Autodesk Fusion 360 part; units mm, degrees
(part 6 of 7)
sketch "Sketch2 (3)" plane through (0, 0, 43) normal (0, 0, 1) x (1, 0, 0) in component "CT idler 3"
  line L0 (67.7594, -49.5331) -> (68.0506, -49.5022)
  line L1 (68.0506, -49.5022) -> (68.1287, -49.4822)
  line L2 (68.1287, -49.4822) -> (68.2056, -49.4521)
  line L3 (68.2056, -49.4521) -> (68.2815, -49.4151)
  line L4 (68.2815, -49.4151) -> (68.3564, -49.3722)
  line L5 (68.3564, -49.3722) -> (68.4303, -49.324)
  line L6 (68.4303, -49.324) -> (68.503, -49.2708)
  line L7 (68.503, -49.2708) -> (68.5745, -49.213)
  line L8 (68.5745, -49.213) -> (68.6447, -49.1507)
  line L9 (68.6447, -49.1507) -> (68.7135, -49.0841)
  line L10 (68.7135, -49.0841) -> (68.7807, -49.0133)
  line L11 (68.7807, -49.0133) -> (68.8462, -48.9384)
  line L12 (68.8462, -48.9384) -> (68.91, -48.8596)
  line L13 (68.91, -48.8596) -> (68.8895, -48.7768)
  line L14 (68.8895, -48.7768) -> (68.8675, -48.6944)
  line L15 (68.8675, -48.6944) -> (68.8438, -48.6125)
  line L16 (68.8438, -48.6125) -> (68.7491, -48.5761)
  line L17 (68.7491, -48.5761) -> (68.6549, -48.5441)
  line L18 (68.6549, -48.5441) -> (68.5613, -48.5164)
  line L19 (68.5613, -48.5164) -> (68.4685, -48.493)
  line L20 (68.4685, -48.493) -> (68.3765, -48.4742)
  line L21 (68.3765, -48.4742) -> (68.2857, -48.4598)
  line L22 (68.2857, -48.4598) -> (68.1961, -48.4502)
  line L23 (68.1961, -48.4502) -> (68.108, -48.4454)
  line L24 (68.108, -48.4454) -> (68.0217, -48.4457)
  line L25 (68.0217, -48.4457) -> (67.9375, -48.4516)
  line L26 (67.9375, -48.4516) -> (67.8559, -48.464)
  line L27 (67.8559, -48.464) -> (67.7783, -48.4857)
  line L28 (67.7783, -48.4857) -> (67.5106, -48.6046)
  line L29 (67.5106, -48.6046) -> (67.4404, -48.4572)
  line L30 (67.4404, -48.4572) -> (67.3626, -48.3138)
  line L31 (67.3626, -48.3138) -> (67.2773, -48.1747)
  line L32 (67.2773, -48.1747) -> (67.1848, -48.0403)
  line L33 (67.1848, -48.0403) -> (67.4216, -47.868)
  line L34 (67.4216, -47.868) -> (67.4792, -47.8116)
  line L35 (67.4792, -47.8116) -> (67.5307, -47.7471)
  line L36 (67.5307, -47.7471) -> (67.578, -47.6771)
  line L37 (67.578, -47.6771) -> (67.6214, -47.6025)
  line L38 (67.6214, -47.6025) -> (67.6613, -47.5238)
  line L39 (67.6613, -47.5238) -> (67.6977, -47.4414)
  line L40 (67.6977, -47.4414) -> (67.7307, -47.3556)
  line L41 (67.7307, -47.3556) -> (67.7603, -47.2665)
  line L42 (67.7603, -47.2665) -> (67.7866, -47.1744)
  line L43 (67.7866, -47.1744) -> (67.8094, -47.0795)
  line L44 (67.8094, -47.0795) -> (67.8287, -46.9819)
  line L45 (67.8287, -46.9819) -> (67.8446, -46.8818)
  line L46 (67.8446, -46.8818) -> (67.7854, -46.8203)
  line L47 (67.7854, -46.8203) -> (67.7251, -46.76)
  line L48 (67.7251, -46.76) -> (67.6636, -46.7009)
  line L49 (67.6636, -46.7009) -> (67.5635, -46.7167)
  line L50 (67.5635, -46.7167) -> (67.4659, -46.736)
  line L51 (67.4659, -46.736) -> (67.371, -46.7588)
  line L52 (67.371, -46.7588) -> (67.2789, -46.7851)
  line L53 (67.2789, -46.7851) -> (67.1899, -46.8147)
  line L54 (67.1899, -46.8147) -> (67.104, -46.8477)
  line L55 (67.104, -46.8477) -> (67.0216, -46.8841)
  line L56 (67.0216, -46.8841) -> (66.9429, -46.924)
  line L57 (66.9429, -46.924) -> (66.8683, -46.9674)
  line L58 (66.8683, -46.9674) -> (66.7983, -47.0147)
  line L59 (66.7983, -47.0147) -> (66.7338, -47.0662)
  line L60 (66.7338, -47.0662) -> (66.6775, -47.1238)
  line L61 (66.6775, -47.1238) -> (66.5051, -47.3606)
  line L62 (66.5051, -47.3606) -> (66.3707, -47.2681)
  line L63 (66.3707, -47.2681) -> (66.2316, -47.1828)
  line L64 (66.2316, -47.1828) -> (66.0882, -47.105)
  line L65 (66.0882, -47.105) -> (65.9409, -47.0348)
  line L66 (65.9409, -47.0348) -> (66.0598, -46.7672)
  line L67 (66.0598, -46.7672) -> (66.0814, -46.6895)
  line L68 (66.0814, -46.6895) -> (66.0938, -46.6079)
  line L69 (66.0938, -46.6079) -> (66.0997, -46.5237)
  line L70 (66.0997, -46.5237) -> (66.1001, -46.4374)
  line L71 (66.1001, -46.4374) -> (66.0952, -46.3493)
  line L72 (66.0952, -46.3493) -> (66.0856, -46.2597)
  line L73 (66.0856, -46.2597) -> (66.0712, -46.1689)
  line L74 (66.0712, -46.1689) -> (66.0524, -46.0769)
  line L75 (66.0524, -46.0769) -> (66.0291, -45.9841)
  line L76 (66.0291, -45.9841) -> (66.0013, -45.8905)
  line L77 (66.0013, -45.8905) -> (65.9693, -45.7963)
  line L78 (65.9693, -45.7963) -> (65.9329, -45.7016)
  line L79 (65.9329, -45.7016) -> (65.851, -45.678)
  line L80 (65.851, -45.678) -> (65.7686, -45.6559)
  line L81 (65.7686, -45.6559) -> (65.6858, -45.6354)
  line L82 (65.6858, -45.6354) -> (65.607, -45.6992)
  line L83 (65.607, -45.6992) -> (65.5321, -45.7648)
  line L84 (65.5321, -45.7648) -> (65.4614, -45.832)
  line L85 (65.4614, -45.832) -> (65.3947, -45.9007)
  line L86 (65.3947, -45.9007) -> (65.3324, -45.9709)
  line L87 (65.3324, -45.9709) -> (65.2746, -46.0424)
  line L88 (65.2746, -46.0424) -> (65.2214, -46.1152)
  line L89 (65.2214, -46.1152) -> (65.1732, -46.189)
  line L90 (65.1732, -46.189) -> (65.1303, -46.2639)
  line L91 (65.1303, -46.2639) -> (65.0933, -46.3398)
  line L92 (65.0933, -46.3398) -> (65.0633, -46.4167)
  line L93 (65.0633, -46.4167) -> (65.0432, -46.4948)
  line L94 (65.0432, -46.4948) -> (65.0123, -46.786)
  line L95 (65.0123, -46.786) -> (64.8497, -46.7731)
  line L96 (64.8497, -46.7731) -> (64.6866, -46.7688)
  line L97 (64.6866, -46.7688) -> (64.5235, -46.7731)
  line L98 (64.5235, -46.7731) -> (64.3608, -46.786)
  line L99 (64.3608, -46.786) -> (64.33, -46.4948)
  line L100 (64.33, -46.4948) -> (64.3099, -46.4167)
  line L101 (64.3099, -46.4167) -> (64.2798, -46.3398)
  line L102 (64.2798, -46.3398) -> (64.2428, -46.2639)
  line L103 (64.2428, -46.2639) -> (64.2, -46.189)
  line L104 (64.2, -46.189) -> (64.1517, -46.1152)
  line L105 (64.1517, -46.1152) -> (64.0986, -46.0424)
  line L106 (64.0986, -46.0424) -> (64.0408, -45.9709)
  line L107 (64.0408, -45.9709) -> (63.9784, -45.9007)
  line L108 (63.9784, -45.9007) -> (63.9118, -45.832)
  line L109 (63.9118, -45.832) -> (63.841, -45.7648)
  line L110 (63.841, -45.7648) -> (63.7662, -45.6992)
  line L111 (63.7662, -45.6992) -> (63.6874, -45.6354)
  line L112 (63.6874, -45.6354) -> (63.6046, -45.6559)
  line L113 (63.6046, -45.6559) -> (63.5222, -45.678)
  line L114 (63.5222, -45.678) -> (63.4402, -45.7016)
  line L115 (63.4402, -45.7016) -> (63.4039, -45.7963)
  line L116 (63.4039, -45.7963) -> (63.3718, -45.8905)
  line L117 (63.3718, -45.8905) -> (63.3441, -45.9841)
  line L118 (63.3441, -45.9841) -> (63.3208, -46.0769)
  line L119 (63.3208, -46.0769) -> (63.3019, -46.1689)
  line L120 (63.3019, -46.1689) -> (63.2876, -46.2597)
  line L121 (63.2876, -46.2597) -> (63.2779, -46.3493)
  line L122 (63.2779, -46.3493) -> (63.2731, -46.4374)
  line L123 (63.2731, -46.4374) -> (63.2734, -46.5237)
  line L124 (63.2734, -46.5237) -> (63.2793, -46.6079)
  line L125 (63.2793, -46.6079) -> (63.2917, -46.6895)
  line L126 (63.2917, -46.6895) -> (63.3134, -46.7672)
  line L127 (63.3134, -46.7672) -> (63.4323, -47.0348)
  line L128 (63.4323, -47.0348) -> (63.285, -47.105)
  line L129 (63.285, -47.105) -> (63.1416, -47.1828)
  line L130 (63.1416, -47.1828) -> (63.0025, -47.2681)
  line L131 (63.0025, -47.2681) -> (62.8681, -47.3606)
  line L132 (62.8681, -47.3606) -> (62.6957, -47.1238)
  line L133 (62.6957, -47.1238) -> (62.6393, -47.0662)
  line L134 (62.6393, -47.0662) -> (62.5748, -47.0147)
  line L135 (62.5748, -47.0147) -> (62.5048, -46.9674)
  line L136 (62.5048, -46.9674) -> (62.4302, -46.924)
  line L137 (62.4302, -46.924) -> (62.3516, -46.8841)
  line L138 (62.3516, -46.8841) -> (62.2692, -46.8477)
  line L139 (62.2692, -46.8477) -> (62.1833, -46.8147)
  line L140 (62.1833, -46.8147) -> (62.0943, -46.7851)
  line L141 (62.0943, -46.7851) -> (62.0022, -46.7588)
  line L142 (62.0022, -46.7588) -> (61.9073, -46.736)
  line L143 (61.9073, -46.736) -> (61.8097, -46.7167)
  line L144 (61.8097, -46.7167) -> (61.7095, -46.7009)
  line L145 (61.7095, -46.7009) -> (61.648, -46.76)
  line L146 (61.648, -46.76) -> (61.5877, -46.8203)
  line L147 (61.5877, -46.8203) -> (61.5286, -46.8818)
  line L148 (61.5286, -46.8818) -> (61.5445, -46.9819)
  line L149 (61.5445, -46.9819) -> (61.5638, -47.0795)
  line L150 (61.5638, -47.0795) -> (61.5866, -47.1744)
  line L151 (61.5866, -47.1744) -> (61.6128, -47.2665)
  line L152 (61.6128, -47.2665) -> (61.6425, -47.3556)
  line L153 (61.6425, -47.3556) -> (61.6755, -47.4414)
  line L154 (61.6755, -47.4414) -> (61.7119, -47.5238)
  line L155 (61.7119, -47.5238) -> (61.7518, -47.6025)
  line L156 (61.7518, -47.6025) -> (61.7952, -47.6771)
  line L157 (61.7952, -47.6771) -> (61.8424, -47.7471)
  line L158 (61.8424, -47.7471) -> (61.894, -47.8116)
  line L159 (61.894, -47.8116) -> (61.9516, -47.868)
  line L160 (61.9516, -47.868) -> (62.1884, -48.0403)
  line L161 (62.1884, -48.0403) -> (62.0959, -48.1747)
  line L162 (62.0959, -48.1747) -> (62.0106, -48.3138)
  line L163 (62.0106, -48.3138) -> (61.9327, -48.4572)
  line L164 (61.9327, -48.4572) -> (61.8626, -48.6046)
  line L165 (61.8626, -48.6046) -> (61.5949, -48.4857)
  line L166 (61.5949, -48.4857) -> (61.5173, -48.464)
  line L167 (61.5173, -48.464) -> (61.4357, -48.4516)
  line L168 (61.4357, -48.4516) -> (61.3515, -48.4457)
  line L169 (61.3515, -48.4457) -> (61.2651, -48.4454)
  line L170 (61.2651, -48.4454) -> (61.177, -48.4502)
  line L171 (61.177, -48.4502) -> (61.0875, -48.4598)
  line L172 (61.0875, -48.4598) -> (60.9966, -48.4742)
  line L173 (60.9966, -48.4742) -> (60.9047, -48.493)
  line L174 (60.9047, -48.493) -> (60.8118, -48.5164)
  line L175 (60.8118, -48.5164) -> (60.7182, -48.5441)
  line L176 (60.7182, -48.5441) -> (60.624, -48.5761)
  line L177 (60.624, -48.5761) -> (60.5294, -48.6125)
  line L178 (60.5294, -48.6125) -> (60.5057, -48.6944)
  line L179 (60.5057, -48.6944) -> (60.4836, -48.7768)
  line L180 (60.4836, -48.7768) -> (60.4632, -48.8596)
  line L181 (60.4632, -48.8596) -> (60.527, -48.9384)
  line L182 (60.527, -48.9384) -> (60.5925, -49.0133)
  line L183 (60.5925, -49.0133) -> (60.6597, -49.0841)
  line L184 (60.6597, -49.0841) -> (60.7285, -49.1507)
  line L185 (60.7285, -49.1507) -> (60.7987, -49.213)
  line L186 (60.7987, -49.213) -> (60.8702, -49.2708)
  line L187 (60.8702, -49.2708) -> (60.9429, -49.324)
  line L188 (60.9429, -49.324) -> (61.0168, -49.3722)
  line L189 (61.0168, -49.3722) -> (61.0917, -49.4151)
  line L190 (61.0917, -49.4151) -> (61.1676, -49.4521)
  line L191 (61.1676, -49.4521) -> (61.2445, -49.4822)
  line L192 (61.2445, -49.4822) -> (61.3225, -49.5022)
  line L193 (61.3225, -49.5022) -> (61.6138, -49.5331)
  line L194 (61.6138, -49.5331) -> (61.6009, -49.6957)
  line L195 (61.6009, -49.6957) -> (61.5966, -49.8588)
  line L196 (61.5966, -49.8588) -> (61.6009, -50.0219)
  line L197 (61.6009, -50.0219) -> (61.6138, -50.1846)
  line L198 (61.6138, -50.1846) -> (61.3225, -50.2155)
  line L199 (61.3225, -50.2155) -> (61.2445, -50.2355)
  line L200 (61.2445, -50.2355) -> (61.1676, -50.2656)
  line L201 (61.1676, -50.2656) -> (61.0917, -50.3026)
  line L202 (61.0917, -50.3026) -> (61.0168, -50.3455)
  line L203 (61.0168, -50.3455) -> (60.9429, -50.3937)
  line L204 (60.9429, -50.3937) -> (60.8702, -50.4468)
  line L205 (60.8702, -50.4468) -> (60.7987, -50.5047)
  line L206 (60.7987, -50.5047) -> (60.7285, -50.567)
  line L207 (60.7285, -50.567) -> (60.6597, -50.6336)
  line L208 (60.6597, -50.6336) -> (60.5925, -50.7044)
  line L209 (60.5925, -50.7044) -> (60.527, -50.7792)
  line L210 (60.527, -50.7792) -> (60.4632, -50.858)
  line L211 (60.4632, -50.858) -> (60.4836, -50.9409)
  line L212 (60.4836, -50.9409) -> (60.5057, -51.0232)
  line L213 (60.5057, -51.0232) -> (60.5294, -51.1052)
  line L214 (60.5294, -51.1052) -> (60.624, -51.1415)
  line L215 (60.624, -51.1415) -> (60.7182, -51.1736)
  line L216 (60.7182, -51.1736) -> (60.8118, -51.2013)
  line L217 (60.8118, -51.2013) -> (60.9047, -51.2246)
  line L218 (60.9047, -51.2246) -> (60.9966, -51.2435)
  line L219 (60.9966, -51.2435) -> (61.0875, -51.2578)
  line L220 (61.0875, -51.2578) -> (61.177, -51.2675)
  line L221 (61.177, -51.2675) -> (61.2651, -51.2723)
  line L222 (61.2651, -51.2723) -> (61.3515, -51.272)
  line L223 (61.3515, -51.272) -> (61.4357, -51.2661)
  line L224 (61.4357, -51.2661) -> (61.5173, -51.2537)
  line L225 (61.5173, -51.2537) -> (61.5949, -51.232)
  line L226 (61.5949, -51.232) -> (61.8626, -51.1131)
  line L227 (61.8626, -51.1131) -> (61.9327, -51.2604)
  line L228 (61.9327, -51.2604) -> (62.0106, -51.4038)
  line L229 (62.0106, -51.4038) -> (62.0959, -51.5429)
  line L230 (62.0959, -51.5429) -> (62.1884, -51.6773)
  line L231 (62.1884, -51.6773) -> (61.9516, -51.8497)
  line L232 (61.9516, -51.8497) -> (61.894, -51.9061)
  line L233 (61.894, -51.9061) -> (61.8424, -51.9706)
  line L234 (61.8424, -51.9706) -> (61.7952, -52.0406)
  line L235 (61.7952, -52.0406) -> (61.7518, -52.1152)
  line L236 (61.7518, -52.1152) -> (61.7119, -52.1939)
  line L237 (61.7119, -52.1939) -> (61.6755, -52.2763)
  line L238 (61.6755, -52.2763) -> (61.6425, -52.3621)
  line L239 (61.6425, -52.3621) -> (61.6128, -52.4512)
  line L240 (61.6128, -52.4512) -> (61.5866, -52.5432)
  line L241 (61.5866, -52.5432) -> (61.5638, -52.6381)
  line L242 (61.5638, -52.6381) -> (61.5445, -52.7357)
  line L243 (61.5445, -52.7357) -> (61.5286, -52.8359)
  line L244 (61.5286, -52.8359) -> (61.5877, -52.8974)
  line L245 (61.5877, -52.8974) -> (61.648, -52.9577)
  line L246 (61.648, -52.9577) -> (61.7095, -53.0168)
  line L247 (61.7095, -53.0168) -> (61.8097, -53.001)
  line L248 (61.8097, -53.001) -> (61.9073, -52.9816)
  line L249 (61.9073, -52.9816) -> (62.0022, -52.9588)
  line L250 (62.0022, -52.9588) -> (62.0943, -52.9326)
  line L251 (62.0943, -52.9326) -> (62.1833, -52.903)
  line L252 (62.1833, -52.903) -> (62.2692, -52.8699)
  line L253 (62.2692, -52.8699) -> (62.3516, -52.8335)
  line L254 (62.3516, -52.8335) -> (62.4302, -52.7937)
  line L255 (62.4302, -52.7937) -> (62.5048, -52.7502)
  line L256 (62.5048, -52.7502) -> (62.5748, -52.703)
  line L257 (62.5748, -52.703) -> (62.6393, -52.6514)
  line L258 (62.6393, -52.6514) -> (62.6957, -52.5939)
  line L259 (62.6957, -52.5939) -> (62.8681, -52.3571)
  line L260 (62.8681, -52.3571) -> (63.0025, -52.4496)
  line L261 (63.0025, -52.4496) -> (63.1416, -52.5348)
  line L262 (63.1416, -52.5348) -> (63.285, -52.6127)
  line L263 (63.285, -52.6127) -> (63.4323, -52.6828)
  line L264 (63.4323, -52.6828) -> (63.3134, -52.9505)
  line L265 (63.3134, -52.9505) -> (63.2917, -53.0281)
  line L266 (63.2917, -53.0281) -> (63.2793, -53.1097)
  line L267 (63.2793, -53.1097) -> (63.2734, -53.194)
  line L268 (63.2734, -53.194) -> (63.2731, -53.2803)
  line L269 (63.2731, -53.2803) -> (63.2779, -53.3684)
  line L270 (63.2779, -53.3684) -> (63.2876, -53.4579)
  line L271 (63.2876, -53.4579) -> (63.3019, -53.5488)
  line L272 (63.3019, -53.5488) -> (63.3208, -53.6407)
  line L273 (63.3208, -53.6407) -> (63.3441, -53.7336)
  line L274 (63.3441, -53.7336) -> (63.3718, -53.8272)
  line L275 (63.3718, -53.8272) -> (63.4039, -53.9214)
  line L276 (63.4039, -53.9214) -> (63.4402, -54.016)
  line L277 (63.4402, -54.016) -> (63.5222, -54.0397)
  line L278 (63.5222, -54.0397) -> (63.6046, -54.0618)
  line L279 (63.6046, -54.0618) -> (63.6874, -54.0822)
  line L280 (63.6874, -54.0822) -> (63.7662, -54.0185)
  line L281 (63.7662, -54.0185) -> (63.841, -53.9529)
  line L282 (63.841, -53.9529) -> (63.9118, -53.8857)
  line L283 (63.9118, -53.8857) -> (63.9784, -53.8169)
  line L284 (63.9784, -53.8169) -> (64.0408, -53.7468)
  line L285 (64.0408, -53.7468) -> (64.0986, -53.6752)
  line L286 (64.0986, -53.6752) -> (64.1517, -53.6025)
  line L287 (64.1517, -53.6025) -> (64.2, -53.5286)
  line L288 (64.2, -53.5286) -> (64.2428, -53.4537)
  line L289 (64.2428, -53.4537) -> (64.2798, -53.3778)
  line L290 (64.2798, -53.3778) -> (64.3099, -53.3009)
  line L291 (64.3099, -53.3009) -> (64.33, -53.2229)
  line L292 (64.33, -53.2229) -> (64.3608, -52.9316)
  line L293 (64.3608, -52.9316) -> (64.5235, -52.9445)
  line L294 (64.5235, -52.9445) -> (64.6866, -52.9488)
  line L295 (64.6866, -52.9488) -> (64.8497, -52.9445)
  line L296 (64.8497, -52.9445) -> (65.0123, -52.9316)
  line L297 (65.0123, -52.9316) -> (65.0432, -53.2229)
  line L298 (65.0432, -53.2229) -> (65.0633, -53.3009)
  line L299 (65.0633, -53.3009) -> (65.0933, -53.3778)
  line L300 (65.0933, -53.3778) -> (65.1303, -53.4537)
  line L301 (65.1303, -53.4537) -> (65.1732, -53.5286)
  line L302 (65.1732, -53.5286) -> (65.2214, -53.6025)
  line L303 (65.2214, -53.6025) -> (65.2746, -53.6752)
  line L304 (65.2746, -53.6752) -> (65.3324, -53.7468)
  line L305 (65.3324, -53.7468) -> (65.3947, -53.8169)
  line L306 (65.3947, -53.8169) -> (65.4614, -53.8857)
  line L307 (65.4614, -53.8857) -> (65.5321, -53.9529)
  line L308 (65.5321, -53.9529) -> (65.607, -54.0185)
  line L309 (65.607, -54.0185) -> (65.6858, -54.0822)
  line L310 (65.6858, -54.0822) -> (65.7686, -54.0618)
  line L311 (65.7686, -54.0618) -> (65.851, -54.0397)
  line L312 (65.851, -54.0397) -> (65.9329, -54.016)
  line L313 (65.9329, -54.016) -> (65.9693, -53.9214)
  line L314 (65.9693, -53.9214) -> (66.0013, -53.8272)
  line L315 (66.0013, -53.8272) -> (66.0291, -53.7336)
  line L316 (66.0291, -53.7336) -> (66.0524, -53.6407)
  line L317 (66.0524, -53.6407) -> (66.0712, -53.5488)
  line L318 (66.0712, -53.5488) -> (66.0856, -53.4579)
  line L319 (66.0856, -53.4579) -> (66.0952, -53.3684)
  line L320 (66.0952, -53.3684) -> (66.1001, -53.2803)
  line L321 (66.1001, -53.2803) -> (66.0997, -53.194)
  line L322 (66.0997, -53.194) -> (66.0938, -53.1097)
  line L323 (66.0938, -53.1097) -> (66.0814, -53.0281)
  line L324 (66.0814, -53.0281) -> (66.0598, -52.9505)
  line L325 (66.0598, -52.9505) -> (65.9409, -52.6828)
  line L326 (65.9409, -52.6828) -> (66.0882, -52.6127)
  line L327 (66.0882, -52.6127) -> (66.2316, -52.5348)
  line L328 (66.2316, -52.5348) -> (66.3707, -52.4496)
  line L329 (66.3707, -52.4496) -> (66.5051, -52.3571)
  line L330 (66.5051, -52.3571) -> (66.6775, -52.5939)
  line L331 (66.6775, -52.5939) -> (66.7338, -52.6514)
  line L332 (66.7338, -52.6514) -> (66.7983, -52.703)
  line L333 (66.7983, -52.703) -> (66.8683, -52.7502)
  line L334 (66.8683, -52.7502) -> (66.9429, -52.7937)
  line L335 (66.9429, -52.7937) -> (67.0216, -52.8335)
  line L336 (67.0216, -52.8335) -> (67.104, -52.8699)
  line L337 (67.104, -52.8699) -> (67.1899, -52.903)
  line L338 (67.1899, -52.903) -> (67.2789, -52.9326)
  line L339 (67.2789, -52.9326) -> (67.371, -52.9588)
  line L340 (67.371, -52.9588) -> (67.4659, -52.9816)
  line L341 (67.4659, -52.9816) -> (67.5635, -53.001)
  line L342 (67.5635, -53.001) -> (67.6636, -53.0168)
  line L343 (67.6636, -53.0168) -> (67.7251, -52.9577)
  line L344 (67.7251, -52.9577) -> (67.7854, -52.8974)
  line L345 (67.7854, -52.8974) -> (67.8446, -52.8359)
  line L346 (67.8446, -52.8359) -> (67.8287, -52.7357)
  line L347 (67.8287, -52.7357) -> (67.8094, -52.6381)
  line L348 (67.8094, -52.6381) -> (67.7866, -52.5432)
  line L349 (67.7866, -52.5432) -> (67.7603, -52.4512)
  line L350 (67.7603, -52.4512) -> (67.7307, -52.3621)
  line L351 (67.7307, -52.3621) -> (67.6977, -52.2763)
  line L352 (67.6977, -52.2763) -> (67.6613, -52.1939)
  line L353 (67.6613, -52.1939) -> (67.6214, -52.1152)
  line L354 (67.6214, -52.1152) -> (67.578, -52.0406)
  line L355 (67.578, -52.0406) -> (67.5307, -51.9706)
  line L356 (67.5307, -51.9706) -> (67.4792, -51.9061)
  line L357 (67.4792, -51.9061) -> (67.4216, -51.8497)
  line L358 (67.4216, -51.8497) -> (67.1848, -51.6773)
  line L359 (67.1848, -51.6773) -> (67.2773, -51.5429)
  line L360 (67.2773, -51.5429) -> (67.3626, -51.4038)
  line L361 (67.3626, -51.4038) -> (67.4404, -51.2604)
  line L362 (67.4404, -51.2604) -> (67.5106, -51.1131)
  line L363 (67.5106, -51.1131) -> (67.7783, -51.232)
  line L364 (67.7783, -51.232) -> (67.8559, -51.2537)
  line L365 (67.8559, -51.2537) -> (67.9375, -51.2661)
  line L366 (67.9375, -51.2661) -> (68.0217, -51.272)
  line L367 (68.0217, -51.272) -> (68.108, -51.2723)
  line L368 (68.108, -51.2723) -> (68.1961, -51.2675)
  line L369 (68.1961, -51.2675) -> (68.2857, -51.2578)
  line L370 (68.2857, -51.2578) -> (68.3765, -51.2435)
  line L371 (68.3765, -51.2435) -> (68.4685, -51.2246)
  line L372 (68.4685, -51.2246) -> (68.5613, -51.2013)
  line L373 (68.5613, -51.2013) -> (68.6549, -51.1736)
  line L374 (68.6549, -51.1736) -> (68.7491, -51.1415)
  line L375 (68.7491, -51.1415) -> (68.8438, -51.1052)
  line L376 (68.8438, -51.1052) -> (68.8675, -51.0232)
  line L377 (68.8675, -51.0232) -> (68.8895, -50.9409)
  line L378 (68.8895, -50.9409) -> (68.91, -50.858)
  line L379 (68.91, -50.858) -> (68.8462, -50.7792)
  line L380 (68.8462, -50.7792) -> (68.7807, -50.7044)
  line L381 (68.7807, -50.7044) -> (68.7135, -50.6336)
  line L382 (68.7135, -50.6336) -> (68.6447, -50.567)
  line L383 (68.6447, -50.567) -> (68.5745, -50.5047)
  line L384 (68.5745, -50.5047) -> (68.503, -50.4468)
  line L385 (68.503, -50.4468) -> (68.4303, -50.3937)
  line L386 (68.4303, -50.3937) -> (68.3564, -50.3455)
  line L387 (68.3564, -50.3455) -> (68.2815, -50.3026)
  line L388 (68.2815, -50.3026) -> (68.2056, -50.2656)
  line L389 (68.2056, -50.2656) -> (68.1287, -50.2355)
  line L390 (68.1287, -50.2355) -> (68.0506, -50.2155)
  line L391 (68.0506, -50.2155) -> (67.7594, -50.1846)
  line L392 (67.7594, -50.1846) -> (67.7723, -50.0219)
  line L393 (67.7723, -50.0219) -> (67.7766, -49.8588)
  line L394 (67.7766, -49.8588) -> (67.7723, -49.6957)
  line L395 (67.7723, -49.6957) -> (67.7594, -49.5331)
extrude "Extrude2''" add sketch "Sketch2 (3)" along normal blind 2.4 separate body makes body 7 in component "CT idler 3"
combine "Combine1''" operation add target body 6 tool bodies 7 in component "CT idler 3"
ref_plane "WorkPlane3" through (0, 0, 41.2) normal (0, 0, 1) x (1, 0, 0) in component "CT idler 3"
sketch "Sketch3 (3)" plane through (0, 0, 41.2) normal (0, 0, 1) x (1, 0, 0) in component "CT idler 3"
  circle A0 centre (64.6866, -49.8588) radius 1.7
extrude "Extrude3''" cut sketch "Sketch3 (3)" along normal blind 4.2 bodies 6 in component "CT idler 3"
ref_plane "WorkPlane1" through (0, 0, 43.4) normal (0, 0, 1) x (1, 0, 0) in component "CT dial wheel (tool body)"
sketch "Sketch1 (5)" plane through (0, 0, 43.4) normal (0, 0, 1) x (1, 0, 0) in component "CT dial wheel (tool body)"
  line L0 (70.4894, -54.5349) -> (70.5857, -54.2102)
  line L1 (70.5857, -54.2102) -> (70.6022, -54.1307)
  line L2 (70.6022, -54.1307) -> (70.6131, -54.0495)
  line L3 (70.6131, -54.0495) -> (70.6203, -53.9673)
  line L4 (70.6203, -53.9673) -> (70.6245, -53.8842)
  line L5 (70.6245, -53.8842) -> (70.6261, -53.8004)
  line L6 (70.6261, -53.8004) -> (70.6251, -53.7159)
  line L7 (70.6251, -53.7159) -> (70.6219, -53.6308)
  line L8 (70.6219, -53.6308) -> (70.6165, -53.5452)
  line L9 (70.6165, -53.5452) -> (70.6091, -53.4591)
  line L10 (70.6091, -53.4591) -> (70.5997, -53.3725)
  line L11 (70.5997, -53.3725) -> (70.5884, -53.2855)
  line L12 (70.5884, -53.2855) -> (70.5752, -53.1981)
  line L13 (70.5752, -53.1981) -> (70.4387, -53.1625)
  line L14 (70.4387, -53.1625) -> (70.3017, -53.1286)
  line L15 (70.3017, -53.1286) -> (70.1643, -53.0965)
  line L16 (70.1643, -53.0965) -> (70.1119, -53.1677)
  line L17 (70.1119, -53.1677) -> (70.0614, -53.2393)
  line L18 (70.0614, -53.2393) -> (70.0127, -53.3115)
  line L19 (70.0127, -53.3115) -> (69.966, -53.3843)
  line L20 (69.966, -53.3843) -> (69.9213, -53.4575)
  line L21 (69.9213, -53.4575) -> (69.8788, -53.5313)
  line L22 (69.8788, -53.5313) -> (69.8386, -53.6056)
  line L23 (69.8386, -53.6056) -> (69.8009, -53.6804)
  line L24 (69.8009, -53.6804) -> (69.7658, -53.7559)
  line L25 (69.7658, -53.7559) -> (69.7339, -53.832)
  line L26 (69.7339, -53.832) -> (69.7057, -53.9089)
  line L27 (69.7057, -53.9089) -> (69.6832, -53.987)
  line L28 (69.6832, -53.987) -> (69.617, -54.3191)
  line L29 (69.617, -54.3191) -> (69.4173, -54.2815)
  line L30 (69.4173, -54.2815) -> (69.2167, -54.248)
  line L31 (69.2167, -54.248) -> (69.0156, -54.2186)
  line L32 (69.0156, -54.2186) -> (68.8139, -54.1934)
  line L33 (68.8139, -54.1934) -> (68.8523, -53.857)
  line L34 (68.8523, -53.857) -> (68.8547, -53.7758)
  line L35 (68.8547, -53.7758) -> (68.8514, -53.6939)
  line L36 (68.8514, -53.6939) -> (68.8442, -53.6117)
  line L37 (68.8442, -53.6117) -> (68.8339, -53.5291)
  line L38 (68.8339, -53.5291) -> (68.8209, -53.4463)
  line L39 (68.8209, -53.4463) -> (68.8053, -53.3633)
  line L40 (68.8053, -53.3633) -> (68.7874, -53.28)
  line L41 (68.7874, -53.28) -> (68.7672, -53.1966)
  line L42 (68.7672, -53.1966) -> (68.7449, -53.1131)
  line L43 (68.7449, -53.1131) -> (68.7206, -53.0295)
  line L44 (68.7206, -53.0295) -> (68.6944, -52.9458)
  line L45 (68.6944, -52.9458) -> (68.6662, -52.8621)
  line L46 (68.6662, -52.8621) -> (68.5256, -52.8507)
  line L47 (68.5256, -52.8507) -> (68.3848, -52.8411)
  line L48 (68.3848, -52.8411) -> (68.2439, -52.8333)
  line L49 (68.2439, -52.8333) -> (68.2047, -52.9125)
  line L50 (68.2047, -52.9125) -> (68.1674, -52.9919)
  line L51 (68.1674, -52.9919) -> (68.132, -53.0714)
  line L52 (68.132, -53.0714) -> (68.0986, -53.1511)
  line L53 (68.0986, -53.1511) -> (68.0673, -53.231)
  line L54 (68.0673, -53.231) -> (68.0382, -53.311)
  line L55 (68.0382, -53.311) -> (68.0116, -53.3912)
  line L56 (68.0116, -53.3912) -> (67.9874, -53.4715)
  line L57 (67.9874, -53.4715) -> (67.966, -53.5519)
  line L58 (67.966, -53.5519) -> (67.9478, -53.6324)
  line L59 (67.9478, -53.6324) -> (67.9334, -53.713)
  line L60 (67.9334, -53.713) -> (67.9248, -53.7938)
  line L61 (67.9248, -53.7938) -> (67.9173, -54.1324)
  line L62 (67.9173, -54.1324) -> (67.714, -54.13)
  line L63 (67.714, -54.13) -> (67.5107, -54.1318)
  line L64 (67.5107, -54.1318) -> (67.3075, -54.1379)
  line L65 (67.3075, -54.1379) -> (67.1045, -54.1481)
  line L66 (67.1045, -54.1481) -> (67.0839, -53.81)
  line L67 (67.0839, -53.81) -> (67.0722, -53.7297)
  line L68 (67.0722, -53.7297) -> (67.0547, -53.6496)
  line L69 (67.0547, -53.6496) -> (67.0334, -53.5699)
  line L70 (67.0334, -53.5699) -> (67.0089, -53.4904)
  line L71 (67.0089, -53.4904) -> (66.9816, -53.4111)
  line L72 (66.9816, -53.4111) -> (66.9519, -53.332)
  line L73 (66.9519, -53.332) -> (66.9197, -53.2532)
  line L74 (66.9197, -53.2532) -> (66.8854, -53.1745)
  line L75 (66.8854, -53.1745) -> (66.849, -53.0962)
  line L76 (66.849, -53.0962) -> (66.8105, -53.018)
  line L77 (66.8105, -53.018) -> (66.7702, -52.9402)
  line L78 (66.7702, -52.9402) -> (66.7279, -52.8626)
  line L79 (66.7279, -52.8626) -> (66.5874, -52.8758)
  line L80 (66.5874, -52.8758) -> (66.4471, -52.8908)
  line L81 (66.4471, -52.8908) -> (66.307, -52.9076)
  line L82 (66.307, -52.9076) -> (66.2821, -52.9924)
  line L83 (66.2821, -52.9924) -> (66.2591, -53.077)
  line L84 (66.2591, -53.077) -> (66.2381, -53.1615)
  line L85 (66.2381, -53.1615) -> (66.219, -53.2458)
  line L86 (66.219, -53.2458) -> (66.2021, -53.3299)
  line L87 (66.2021, -53.3299) -> (66.1874, -53.4138)
  line L88 (66.1874, -53.4138) -> (66.175, -53.4974)
  line L89 (66.175, -53.4974) -> (66.1652, -53.5806)
  line L90 (66.1652, -53.5806) -> (66.1581, -53.6635)
  line L91 (66.1581, -53.6635) -> (66.1541, -53.746)
  line L92 (66.1541, -53.746) -> (66.154, -53.8279)
  line L93 (66.154, -53.8279) -> (66.1595, -53.9089)
  line L94 (66.1595, -53.9089) -> (66.2109, -54.2437)
  line L95 (66.2109, -54.2437) -> (66.0103, -54.2766)
  line L96 (66.0103, -54.2766) -> (65.8104, -54.3137)
  line L97 (65.8104, -54.3137) -> (65.6113, -54.3549)
  line L98 (65.6113, -54.3549) -> (65.4132, -54.4003)
  line L99 (65.4132, -54.4003) -> (65.3342, -54.0709)
  line L100 (65.3342, -54.0709) -> (65.3087, -53.9938)
  line L101 (65.3087, -53.9938) -> (65.2776, -53.918)
  line L102 (65.2776, -53.918) -> (65.2427, -53.8432)
  line L103 (65.2427, -53.8432) -> (65.2048, -53.7691)
  line L104 (65.2048, -53.7691) -> (65.1642, -53.6958)
  line L105 (65.1642, -53.6958) -> (65.1212, -53.6231)
  line L106 (65.1212, -53.6231) -> (65.0759, -53.551)
  line L107 (65.0759, -53.551) -> (65.0284, -53.4795)
  line L108 (65.0284, -53.4795) -> (64.9789, -53.4087)
  line L109 (64.9789, -53.4087) -> (64.9275, -53.3384)
  line L110 (64.9275, -53.3384) -> (64.8742, -53.2688)
  line L111 (64.8742, -53.2688) -> (64.8191, -53.1997)
  line L112 (64.8191, -53.1997) -> (64.683, -53.2371)
  line L113 (64.683, -53.2371) -> (64.5475, -53.2762)
  line L114 (64.5475, -53.2762) -> (64.4124, -53.3171)
  line L115 (64.4124, -53.3171) -> (64.4026, -53.4049)
  line L116 (64.4026, -53.4049) -> (64.3947, -53.4923)
  line L117 (64.3947, -53.4923) -> (64.3886, -53.5791)
  line L118 (64.3886, -53.5791) -> (64.3845, -53.6655)
  line L119 (64.3845, -53.6655) -> (64.3825, -53.7512)
  line L120 (64.3825, -53.7512) -> (64.3825, -53.8364)
  line L121 (64.3825, -53.8364) -> (64.3849, -53.9208)
  line L122 (64.3849, -53.9208) -> (64.3896, -54.0045)
  line L123 (64.3896, -54.0045) -> (64.397, -54.0874)
  line L124 (64.397, -54.0874) -> (64.4074, -54.1693)
  line L125 (64.4074, -54.1693) -> (64.4215, -54.25)
  line L126 (64.4215, -54.25) -> (64.441, -54.3288)
  line L127 (64.441, -54.3288) -> (64.5498, -54.6496)
  line L128 (64.5498, -54.6496) -> (64.3579, -54.7168)
  line L129 (64.3579, -54.7168) -> (64.1675, -54.7881)
  line L130 (64.1675, -54.7881) -> (63.9786, -54.8632)
  line L131 (63.9786, -54.8632) -> (63.7913, -54.9423)
  line L132 (63.7913, -54.9423) -> (63.6564, -54.6317)
  line L133 (63.6564, -54.6317) -> (63.6179, -54.5602)
  line L134 (63.6179, -54.5602) -> (63.5741, -54.491)
  line L135 (63.5741, -54.491) -> (63.5268, -54.4233)
  line L136 (63.5268, -54.4233) -> (63.4766, -54.3569)
  line L137 (63.4766, -54.3569) -> (63.4239, -54.2917)
  line L138 (63.4239, -54.2917) -> (63.3688, -54.2276)
  line L139 (63.3688, -54.2276) -> (63.3117, -54.1645)
  line L140 (63.3117, -54.1645) -> (63.2525, -54.1024)
  line L141 (63.2525, -54.1024) -> (63.1915, -54.0412)
  line L142 (63.1915, -54.0412) -> (63.1287, -53.9809)
  line L143 (63.1287, -53.9809) -> (63.0641, -53.9216)
  line L144 (63.0641, -53.9216) -> (62.9978, -53.8631)
  line L145 (62.9978, -53.8631) -> (62.8703, -53.9236)
  line L146 (62.8703, -53.9236) -> (62.7436, -53.9857)
  line L147 (62.7436, -53.9857) -> (62.6177, -54.0494)
  line L148 (62.6177, -54.0494) -> (62.6233, -54.1375)
  line L149 (62.6233, -54.1375) -> (62.6307, -54.225)
  line L150 (62.6307, -54.225) -> (62.6398, -54.3115)
  line L151 (62.6398, -54.3115) -> (62.6507, -54.3973)
  line L152 (62.6507, -54.3973) -> (62.6636, -54.4821)
  line L153 (62.6636, -54.4821) -> (62.6785, -54.5659)
  line L154 (62.6785, -54.5659) -> (62.6954, -54.6487)
  line L155 (62.6954, -54.6487) -> (62.7146, -54.7303)
  line L156 (62.7146, -54.7303) -> (62.7363, -54.8106)
  line L157 (62.7363, -54.8106) -> (62.7608, -54.8895)
  line L158 (62.7608, -54.8895) -> (62.7886, -54.9665)
  line L159 (62.7886, -54.9665) -> (62.8216, -55.0408)
  line L160 (62.8216, -55.0408) -> (62.9844, -55.3377)
  line L161 (62.9844, -55.3377) -> (62.8071, -55.4373)
  line L162 (62.8071, -55.4373) -> (62.632, -55.5405)
  line L163 (62.632, -55.5405) -> (62.459, -55.6473)
  line L164 (62.459, -55.6473) -> (62.2883, -55.7577)
  line L165 (62.2883, -55.7577) -> (62.1015, -55.4752)
  line L166 (62.1015, -55.4752) -> (62.0511, -55.4115)
  line L167 (62.0511, -55.4115) -> (61.9959, -55.351)
  line L168 (61.9959, -55.351) -> (61.9376, -55.2926)
  line L169 (61.9376, -55.2926) -> (61.8767, -55.2359)
  line L170 (61.8767, -55.2359) -> (61.8134, -55.1809)
  line L171 (61.8134, -55.1809) -> (61.7481, -55.1273)
  line L172 (61.7481, -55.1273) -> (61.6809, -55.0751)
  line L173 (61.6809, -55.0751) -> (61.6118, -55.0241)
  line L174 (61.6118, -55.0241) -> (61.5411, -54.9745)
  line L175 (61.5411, -54.9745) -> (61.4687, -54.926)
  line L176 (61.4687, -54.926) -> (61.3948, -54.8788)
  line L177 (61.3948, -54.8788) -> (61.3194, -54.8327)
  line L178 (61.3194, -54.8327) -> (61.2044, -54.9144)
  line L179 (61.2044, -54.9144) -> (61.0904, -54.9976)
  line L180 (61.0904, -54.9976) -> (60.9774, -55.0821)
  line L181 (60.9774, -55.0821) -> (60.9983, -55.168)
  line L182 (60.9983, -55.168) -> (61.0207, -55.2528)
  line L183 (61.0207, -55.2528) -> (61.0447, -55.3365)
  line L184 (61.0447, -55.3365) -> (61.0704, -55.4191)
  line L185 (61.0704, -55.4191) -> (61.0978, -55.5003)
  line L186 (61.0978, -55.5003) -> (61.127, -55.5803)
  line L187 (61.127, -55.5803) -> (61.158, -55.6589)
  line L188 (61.158, -55.6589) -> (61.1911, -55.7359)
  line L189 (61.1911, -55.7359) -> (61.2264, -55.8113)
  line L190 (61.2264, -55.8113) -> (61.2642, -55.8847)
  line L191 (61.2642, -55.8847) -> (61.305, -55.9557)
  line L192 (61.305, -55.9557) -> (61.3503, -56.0231)
  line L193 (61.3503, -56.0231) -> (61.5622, -56.2873)
  line L194 (61.5622, -56.2873) -> (61.405, -56.4161)
  line L195 (61.405, -56.4161) -> (61.2504, -56.5482)
  line L196 (61.2504, -56.5482) -> (61.0986, -56.6834)
  line L197 (61.0986, -56.6834) -> (60.9497, -56.8218)
  line L198 (60.9497, -56.8218) -> (60.7166, -56.576)
  line L199 (60.7166, -56.576) -> (60.656, -56.522)
  line L200 (60.656, -56.522) -> (60.5911, -56.4719)
  line L201 (60.5911, -56.4719) -> (60.5235, -56.4246)
  line L202 (60.5235, -56.4246) -> (60.4537, -56.3794)
  line L203 (60.4537, -56.3794) -> (60.3818, -56.3361)
  line L204 (60.3818, -56.3361) -> (60.3082, -56.2947)
  line L205 (60.3082, -56.2947) -> (60.2329, -56.2549)
  line L206 (60.2329, -56.2549) -> (60.1561, -56.2168)
  line L207 (60.1561, -56.2168) -> (60.0778, -56.1802)
  line L208 (60.0778, -56.1802) -> (59.9981, -56.145)
  line L209 (59.9981, -56.145) -> (59.9171, -56.1113)
  line L210 (59.9171, -56.1113) -> (59.8349, -56.0791)
  line L211 (59.8349, -56.0791) -> (59.7358, -56.1795)
  line L212 (59.7358, -56.1795) -> (59.638, -56.2812)
  line L213 (59.638, -56.2812) -> (59.5414, -56.3841)
  line L214 (59.5414, -56.3841) -> (59.5769, -56.465)
  line L215 (59.5769, -56.465) -> (59.6136, -56.5447)
  line L216 (59.6136, -56.5447) -> (59.6518, -56.6229)
  line L217 (59.6518, -56.6229) -> (59.6914, -56.6997)
  line L218 (59.6914, -56.6997) -> (59.7325, -56.775)
  line L219 (59.7325, -56.775) -> (59.7752, -56.8487)
  line L220 (59.7752, -56.8487) -> (59.8194, -56.9207)
  line L221 (59.8194, -56.9207) -> (59.8654, -56.9908)
  line L222 (59.8654, -56.9908) -> (59.9132, -57.0589)
  line L223 (59.9132, -57.0589) -> (59.9632, -57.1246)
  line L224 (59.9632, -57.1246) -> (60.0157, -57.1874)
  line L225 (60.0157, -57.1874) -> (60.072, -57.246)
  line L226 (60.072, -57.246) -> (60.3266, -57.4694)
  line L227 (60.3266, -57.4694) -> (60.1941, -57.6235)
  line L228 (60.1941, -57.6235) -> (60.0648, -57.7804)
  line L229 (60.0648, -57.7804) -> (59.9388, -57.94)
  line L230 (59.9388, -57.94) -> (59.8162, -58.1021)
  line L231 (59.8162, -58.1021) -> (59.544, -57.9005)
  line L232 (59.544, -57.9005) -> (59.4749, -57.8579)
  line L233 (59.4749, -57.8579) -> (59.4023, -57.8198)
  line L234 (59.4023, -57.8198) -> (59.3275, -57.7849)
  line L235 (59.3275, -57.7849) -> (59.2509, -57.7525)
  line L236 (59.2509, -57.7525) -> (59.1726, -57.7224)
  line L237 (59.1726, -57.7224) -> (59.0929, -57.6944)
  line L238 (59.0929, -57.6944) -> (59.0119, -57.6683)
  line L239 (59.0119, -57.6683) -> (58.9296, -57.6441)
  line L240 (58.9296, -57.6441) -> (58.8461, -57.6216)
  line L241 (58.8461, -57.6216) -> (58.7616, -57.6009)
  line L242 (58.7616, -57.6009) -> (58.676, -57.5818)
  line L243 (58.676, -57.5818) -> (58.5893, -57.5642)
  line L244 (58.5893, -57.5642) -> (58.5092, -57.6804)
  line L245 (58.5092, -57.6804) -> (58.4305, -57.7975)
  line L246 (58.4305, -57.7975) -> (58.3533, -57.9156)
  line L247 (58.3533, -57.9156) -> (58.4022, -57.9892)
  line L248 (58.4022, -57.9892) -> (58.4523, -58.0612)
  line L249 (58.4523, -58.0612) -> (58.5035, -58.1316)
  line L250 (58.5035, -58.1316) -> (58.5559, -58.2004)
  line L251 (58.5559, -58.2004) -> (58.6094, -58.2674)
  line L252 (58.6094, -58.2674) -> (58.6642, -58.3326)
  line L253 (58.6642, -58.3326) -> (58.7202, -58.3958)
  line L254 (58.7202, -58.3958) -> (58.7777, -58.4569)
  line L255 (58.7777, -58.4569) -> (58.8366, -58.5156)
  line L256 (58.8366, -58.5156) -> (58.8973, -58.5716)
  line L257 (58.8973, -58.5716) -> (58.9599, -58.6244)
  line L258 (58.9599, -58.6244) -> (59.0255, -58.6723)
  line L259 (59.0255, -58.6723) -> (59.315, -58.848)
  line L260 (59.315, -58.848) -> (59.2113, -59.0229)
  line L261 (59.2113, -59.0229) -> (59.1112, -59.1999)
  line L262 (59.1112, -59.1999) -> (59.0148, -59.3788)
  line L263 (59.0148, -59.3788) -> (58.9222, -59.5598)
  line L264 (58.9222, -59.5598) -> (58.6191, -59.4086)
  line L265 (58.6191, -59.4086) -> (58.5437, -59.3786)
  line L266 (58.5437, -59.3786) -> (58.4656, -59.3537)
  line L267 (58.4656, -59.3537) -> (58.3859, -59.3323)
  line L268 (58.3859, -59.3323) -> (58.3048, -59.3137)
  line L269 (58.3048, -59.3137) -> (58.2225, -59.2977)
  line L270 (58.2225, -59.2977) -> (58.1391, -59.2839)
  line L271 (58.1391, -59.2839) -> (58.0548, -59.2723)
  line L272 (58.0548, -59.2723) -> (57.9696, -59.2627)
  line L273 (57.9696, -59.2627) -> (57.8835, -59.2551)
  line L274 (57.8835, -59.2551) -> (57.7966, -59.2493)
  line L275 (57.7966, -59.2493) -> (57.7089, -59.2454)
  line L276 (57.7089, -59.2454) -> (57.6206, -59.2432)
  line L277 (57.6206, -59.2432) -> (57.5618, -59.3714)
  line L278 (57.5618, -59.3714) -> (57.5047, -59.5004)
  line L279 (57.5047, -59.5004) -> (57.4492, -59.6301)
  line L280 (57.4492, -59.6301) -> (57.5101, -59.6941)
  line L281 (57.5101, -59.6941) -> (57.572, -59.7563)
  line L282 (57.572, -59.7563) -> (57.6346, -59.8168)
  line L283 (57.6346, -59.8168) -> (57.6981, -59.8755)
  line L284 (57.6981, -59.8755) -> (57.7625, -59.9322)
  line L285 (57.7625, -59.9322) -> (57.8277, -59.9868)
  line L286 (57.8277, -59.9868) -> (57.8939, -60.0393)
  line L287 (57.8939, -60.0393) -> (57.9611, -60.0895)
  line L288 (57.9611, -60.0895) -> (58.0294, -60.1371)
  line L289 (58.0294, -60.1371) -> (58.0988, -60.1818)
  line L290 (58.0988, -60.1818) -> (58.1696, -60.2229)
  line L291 (58.1696, -60.2229) -> (58.2426, -60.2586)
  line L292 (58.2426, -60.2586) -> (58.5582, -60.3814)
  line L293 (58.5582, -60.3814) -> (58.4864, -60.5716)
  line L294 (58.4864, -60.5716) -> (58.4186, -60.7633)
  line L295 (58.4186, -60.7633) -> (58.3548, -60.9563)
  line L296 (58.3548, -60.9563) -> (58.2949, -61.1506)
  line L297 (58.2949, -61.1506) -> (57.9702, -61.0543)
  line L298 (57.9702, -61.0543) -> (57.8907, -61.0378)
  line L299 (57.8907, -61.0378) -> (57.8095, -61.0269)
  line L300 (57.8095, -61.0269) -> (57.7273, -61.0197)
  line L301 (57.7273, -61.0197) -> (57.6442, -61.0155)
  line L302 (57.6442, -61.0155) -> (57.5604, -61.0139)
  line L303 (57.5604, -61.0139) -> (57.4759, -61.0149)
  line L304 (57.4759, -61.0149) -> (57.3908, -61.0181)
  line L305 (57.3908, -61.0181) -> (57.3052, -61.0235)
  line L306 (57.3052, -61.0235) -> (57.2191, -61.0309)
  line L307 (57.2191, -61.0309) -> (57.1325, -61.0403)
  line L308 (57.1325, -61.0403) -> (57.0455, -61.0516)
  line L309 (57.0455, -61.0516) -> (56.9581, -61.0648)
  line L310 (56.9581, -61.0648) -> (56.9225, -61.2013)
  line L311 (56.9225, -61.2013) -> (56.8886, -61.3383)
  line L312 (56.8886, -61.3383) -> (56.8565, -61.4757)
  line L313 (56.8565, -61.4757) -> (56.9277, -61.5281)
  line L314 (56.9277, -61.5281) -> (56.9993, -61.5786)
  line L315 (56.9993, -61.5786) -> (57.0715, -61.6273)
  line L316 (57.0715, -61.6273) -> (57.1443, -61.674)
  line L317 (57.1443, -61.674) -> (57.2175, -61.7187)
  line L318 (57.2175, -61.7187) -> (57.2913, -61.7612)
  line L319 (57.2913, -61.7612) -> (57.3656, -61.8014)
  line L320 (57.3656, -61.8014) -> (57.4404, -61.8391)
  line L321 (57.4404, -61.8391) -> (57.5159, -61.8742)
  line L322 (57.5159, -61.8742) -> (57.592, -61.9061)
  line L323 (57.592, -61.9061) -> (57.6689, -61.9343)
  line L324 (57.6689, -61.9343) -> (57.747, -61.9568)
  line L325 (57.747, -61.9568) -> (58.0791, -62.023)
  line L326 (58.0791, -62.023) -> (58.0415, -62.2227)
  line L327 (58.0415, -62.2227) -> (58.008, -62.4233)
  line L328 (58.008, -62.4233) -> (57.9786, -62.6244)
  line L329 (57.9786, -62.6244) -> (57.9534, -62.8261)
  line L330 (57.9534, -62.8261) -> (57.617, -62.7877)
  line L331 (57.617, -62.7877) -> (57.5358, -62.7853)
  line L332 (57.5358, -62.7853) -> (57.4539, -62.7886)
  line L333 (57.4539, -62.7886) -> (57.3717, -62.7958)
  line L334 (57.3717, -62.7958) -> (57.2891, -62.8061)
  line L335 (57.2891, -62.8061) -> (57.2063, -62.8191)
  line L336 (57.2063, -62.8191) -> (57.1233, -62.8347)
  line L337 (57.1233, -62.8347) -> (57.04, -62.8526)
  line L338 (57.04, -62.8526) -> (56.9566, -62.8728)
  line L339 (56.9566, -62.8728) -> (56.8731, -62.8951)
  line L340 (56.8731, -62.8951) -> (56.7895, -62.9194)
  line L341 (56.7895, -62.9194) -> (56.7058, -62.9456)
  line L342 (56.7058, -62.9456) -> (56.6221, -62.9738)
  line L343 (56.6221, -62.9738) -> (56.6107, -63.1144)
  line L344 (56.6107, -63.1144) -> (56.6011, -63.2552)
  line L345 (56.6011, -63.2552) -> (56.5933, -63.3961)
  line L346 (56.5933, -63.3961) -> (56.6725, -63.4353)
  line L347 (56.6725, -63.4353) -> (56.7519, -63.4726)
  line L348 (56.7519, -63.4726) -> (56.8314, -63.508)
  line L349 (56.8314, -63.508) -> (56.9111, -63.5414)
  line L350 (56.9111, -63.5414) -> (56.991, -63.5727)
  line L351 (56.991, -63.5727) -> (57.071, -63.6018)
  line L352 (57.071, -63.6018) -> (57.1512, -63.6284)
  line L353 (57.1512, -63.6284) -> (57.2315, -63.6526)
  line L354 (57.2315, -63.6526) -> (57.3119, -63.674)
  line L355 (57.3119, -63.674) -> (57.3924, -63.6922)
  line L356 (57.3924, -63.6922) -> (57.473, -63.7066)
  line L357 (57.473, -63.7066) -> (57.5538, -63.7152)
  line L358 (57.5538, -63.7152) -> (57.8924, -63.7227)
  line L359 (57.8924, -63.7227) -> (57.89, -63.926)
  line L360 (57.89, -63.926) -> (57.8918, -64.1293)
  line L361 (57.8918, -64.1293) -> (57.8979, -64.3325)
  line L362 (57.8979, -64.3325) -> (57.9081, -64.5355)
  line L363 (57.9081, -64.5355) -> (57.57, -64.5561)
  line L364 (57.57, -64.5561) -> (57.4897, -64.5678)
  line L365 (57.4897, -64.5678) -> (57.4096, -64.5853)
  line L366 (57.4096, -64.5853) -> (57.3299, -64.6066)
  line L367 (57.3299, -64.6066) -> (57.2504, -64.6311)
  line L368 (57.2504, -64.6311) -> (57.1711, -64.6584)
  line L369 (57.1711, -64.6584) -> (57.092, -64.6881)
  line L370 (57.092, -64.6881) -> (57.0132, -64.7203)
  line L371 (57.0132, -64.7203) -> (56.9345, -64.7546)
  line L372 (56.9345, -64.7546) -> (56.8562, -64.791)
  line L373 (56.8562, -64.791) -> (56.778, -64.8295)
  line L374 (56.778, -64.8295) -> (56.7002, -64.8698)
  line L375 (56.7002, -64.8698) -> (56.6226, -64.9121)
  line L376 (56.6226, -64.9121) -> (56.6358, -65.0526)
  line L377 (56.6358, -65.0526) -> (56.6508, -65.1929)
  line L378 (56.6508, -65.1929) -> (56.6676, -65.333)
  line L379 (56.6676, -65.333) -> (56.7524, -65.3579)
  line L380 (56.7524, -65.3579) -> (56.837, -65.3809)
  line L381 (56.837, -65.3809) -> (56.9215, -65.4019)
  line L382 (56.9215, -65.4019) -> (57.0058, -65.421)
  line L383 (57.0058, -65.421) -> (57.0899, -65.4379)
  line L384 (57.0899, -65.4379) -> (57.1738, -65.4526)
  line L385 (57.1738, -65.4526) -> (57.2574, -65.465)
  line L386 (57.2574, -65.465) -> (57.3406, -65.4748)
  line L387 (57.3406, -65.4748) -> (57.4235, -65.4819)
  line L388 (57.4235, -65.4819) -> (57.506, -65.4859)
  line L389 (57.506, -65.4859) -> (57.5879, -65.486)
  line L390 (57.5879, -65.486) -> (57.6689, -65.4805)
  line L391 (57.6689, -65.4805) -> (58.0037, -65.4291)
  line L392 (58.0037, -65.4291) -> (58.0366, -65.6297)
  line L393 (58.0366, -65.6297) -> (58.0737, -65.8296)
  line L394 (58.0737, -65.8296) -> (58.1149, -66.0287)
  line L395 (58.1149, -66.0287) -> (58.1603, -66.2268)
  line L396 (58.1603, -66.2268) -> (57.8309, -66.3058)
  line L397 (57.8309, -66.3058) -> (57.7538, -66.3313)
  line L398 (57.7538, -66.3313) -> (57.678, -66.3624)
  line L399 (57.678, -66.3624) -> (57.6032, -66.3973)
  line L400 (57.6032, -66.3973) -> (57.5291, -66.4352)
  line L401 (57.5291, -66.4352) -> (57.4558, -66.4758)
  line L402 (57.4558, -66.4758) -> (57.3831, -66.5188)
  line L403 (57.3831, -66.5188) -> (57.311, -66.5641)
  line L404 (57.311, -66.5641) -> (57.2395, -66.6116)
  line L405 (57.2395, -66.6116) -> (57.1687, -66.6611)
  line L406 (57.1687, -66.6611) -> (57.0984, -66.7125)
  line L407 (57.0984, -66.7125) -> (57.0288, -66.7658)
  line L408 (57.0288, -66.7658) -> (56.9597, -66.8209)
  line L409 (56.9597, -66.8209) -> (56.9971, -66.957)
  line L410 (56.9971, -66.957) -> (57.0362, -67.0925)
  line L411 (57.0362, -67.0925) -> (57.0771, -67.2276)
  line L412 (57.0771, -67.2276) -> (57.1649, -67.2374)
  line L413 (57.1649, -67.2374) -> (57.2523, -67.2453)
  line L414 (57.2523, -67.2453) -> (57.3391, -67.2514)
  line L415 (57.3391, -67.2514) -> (57.4255, -67.2555)
  line L416 (57.4255, -67.2555) -> (57.5112, -67.2575)
  line L417 (57.5112, -67.2575) -> (57.5964, -67.2575)
  line L418 (57.5964, -67.2575) -> (57.6808, -67.2551)
  line L419 (57.6808, -67.2551) -> (57.7645, -67.2504)
  line L420 (57.7645, -67.2504) -> (57.8474, -67.243)
  line L421 (57.8474, -67.243) -> (57.9293, -67.2326)
  line L422 (57.9293, -67.2326) -> (58.01, -67.2185)
  line L423 (58.01, -67.2185) -> (58.0888, -67.199)
  line L424 (58.0888, -67.199) -> (58.4096, -67.0902)
  line L425 (58.4096, -67.0902) -> (58.4768, -67.2821)
  line L426 (58.4768, -67.2821) -> (58.5481, -67.4725)
  line L427 (58.5481, -67.4725) -> (58.6232, -67.6614)
  line L428 (58.6232, -67.6614) -> (58.7023, -67.8487)
  line L429 (58.7023, -67.8487) -> (58.3917, -67.9836)
  line L430 (58.3917, -67.9836) -> (58.3202, -68.0221)
  line L431 (58.3202, -68.0221) -> (58.251, -68.0659)
  line L432 (58.251, -68.0659) -> (58.1833, -68.1132)
  line L433 (58.1833, -68.1132) -> (58.1169, -68.1634)
  line L434 (58.1169, -68.1634) -> (58.0517, -68.2161)
  line L435 (58.0517, -68.2161) -> (57.9876, -68.2712)
  line L436 (57.9876, -68.2712) -> (57.9245, -68.3283)
  line L437 (57.9245, -68.3283) -> (57.8624, -68.3875)
  line L438 (57.8624, -68.3875) -> (57.8012, -68.4485)
  line L439 (57.8012, -68.4485) -> (57.7409, -68.5113)
  line L440 (57.7409, -68.5113) -> (57.6816, -68.5759)
  line L441 (57.6816, -68.5759) -> (57.6231, -68.6422)
  line L442 (57.6231, -68.6422) -> (57.6836, -68.7697)
  line L443 (57.6836, -68.7697) -> (57.7457, -68.8964)
  line L444 (57.7457, -68.8964) -> (57.8094, -69.0223)
  line L445 (57.8094, -69.0223) -> (57.8975, -69.0167)
  line L446 (57.8975, -69.0167) -> (57.985, -69.0093)
  line L447 (57.985, -69.0093) -> (58.0715, -69.0002)
  line L448 (58.0715, -69.0002) -> (58.1573, -68.9893)
  line L449 (58.1573, -68.9893) -> (58.2421, -68.9764)
  line L450 (58.2421, -68.9764) -> (58.3259, -68.9615)
  line L451 (58.3259, -68.9615) -> (58.4087, -68.9446)
  line L452 (58.4087, -68.9446) -> (58.4903, -68.9254)
  line L453 (58.4903, -68.9254) -> (58.5706, -68.9037)
  line L454 (58.5706, -68.9037) -> (58.6495, -68.8792)
  line L455 (58.6495, -68.8792) -> (58.7265, -68.8514)
  line L456 (58.7265, -68.8514) -> (58.8008, -68.8184)
  line L457 (58.8008, -68.8184) -> (59.0977, -68.6556)
  line L458 (59.0977, -68.6556) -> (59.1973, -68.8329)
  line L459 (59.1973, -68.8329) -> (59.3005, -69.008)
  line L460 (59.3005, -69.008) -> (59.4073, -69.181)
  line L461 (59.4073, -69.181) -> (59.5177, -69.3517)
  line L462 (59.5177, -69.3517) -> (59.2352, -69.5385)
  line L463 (59.2352, -69.5385) -> (59.1715, -69.5889)
  line L464 (59.1715, -69.5889) -> (59.111, -69.6441)
  line L465 (59.111, -69.6441) -> (59.0526, -69.7024)
  line L466 (59.0526, -69.7024) -> (58.9959, -69.7633)
  line L467 (58.9959, -69.7633) -> (58.9409, -69.8266)
  line L468 (58.9409, -69.8266) -> (58.8873, -69.8919)
  line L469 (58.8873, -69.8919) -> (58.8351, -69.9591)
  line L470 (58.8351, -69.9591) -> (58.7841, -70.0282)
  line L471 (58.7841, -70.0282) -> (58.7345, -70.0989)
  line L472 (58.7345, -70.0989) -> (58.686, -70.1713)
  line L473 (58.686, -70.1713) -> (58.6388, -70.2452)
  line L474 (58.6388, -70.2452) -> (58.5927, -70.3206)
  line L475 (58.5927, -70.3206) -> (58.6744, -70.4356)
  line L476 (58.6744, -70.4356) -> (58.7576, -70.5496)
  line L477 (58.7576, -70.5496) -> (58.8421, -70.6626)
  line L478 (58.8421, -70.6626) -> (58.928, -70.6417)
  line L479 (58.928, -70.6417) -> (59.0128, -70.6193)
  line L480 (59.0128, -70.6193) -> (59.0965, -70.5953)
  line L481 (59.0965, -70.5953) -> (59.1791, -70.5696)
  line L482 (59.1791, -70.5696) -> (59.2603, -70.5422)
  line L483 (59.2603, -70.5422) -> (59.3403, -70.513)
  line L484 (59.3403, -70.513) -> (59.4189, -70.482)
  line L485 (59.4189, -70.482) -> (59.4959, -70.4489)
  line L486 (59.4959, -70.4489) -> (59.5713, -70.4136)
  line L487 (59.5713, -70.4136) -> (59.6447, -70.3758)
  line L488 (59.6447, -70.3758) -> (59.7157, -70.335)
  line L489 (59.7157, -70.335) -> (59.7831, -70.2897)
  line L490 (59.7831, -70.2897) -> (60.0473, -70.0778)
  line L491 (60.0473, -70.0778) -> (60.1761, -70.235)
  line L492 (60.1761, -70.235) -> (60.3082, -70.3896)
  line L493 (60.3082, -70.3896) -> (60.4434, -70.5414)
  line L494 (60.4434, -70.5414) -> (60.5818, -70.6903)
  line L495 (60.5818, -70.6903) -> (60.336, -70.9234)
  line L496 (60.336, -70.9234) -> (60.282, -70.984)
  line L497 (60.282, -70.984) -> (60.2319, -71.0489)
  line L498 (60.2319, -71.0489) -> (60.1846, -71.1165)
  line L499 (60.1846, -71.1165) -> (60.1394, -71.1863)
  line L500 (60.1394, -71.1863) -> (60.0961, -71.2582)
  line L501 (60.0961, -71.2582) -> (60.0547, -71.3318)
  line L502 (60.0547, -71.3318) -> (60.0149, -71.4071)
  line L503 (60.0149, -71.4071) -> (59.9768, -71.4839)
  line L504 (59.9768, -71.4839) -> (59.9402, -71.5622)
  line L505 (59.9402, -71.5622) -> (59.905, -71.6419)